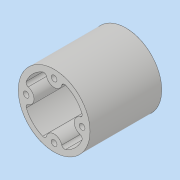
# Autodesk Inventor part: SpoolSmall
Saved by Autodesk Inventor 2017 (Build 210142000, 142)
## iProperties
Created: 2018-04-03
Part Number: SpoolSmall
Material: Generic
Document SubType Name: Modeling
Designer: Derek Wider
Density: 1 g/cm^3
Appearance: Default
Author: Derek Wider
Autodesk Inventor part; units mm, degrees
ref_plane "YZ Plane" through (0, 0, 0) normal (1, 0, 0) x (0, 1, 0)
ref_plane "XZ Plane" through (0, 0, 0) normal (0, 1, 0) x (-1, 0, 0)
ref_plane "XY Plane" through (0, 0, 0) normal (0, 0, 1) x (1, 0, 0)
sketch "Sketch1" plane through (0, 0, 0) normal (0, 0, 1) x (1, 0, 0)
  circle A0 centre (0, 0) radius 15.875
  dimension "d0" = 31.75
  constraints: 1 centre point, 1 coincident
  measures "d0" diameter of A0
extrude "Extrusion1" add sketch "Sketch1" along normal blind 31.75
shell "Shell1" thickness 2.54 removed faces 2 at (-8.4384, -2.4592, 31.75) at (-8.4384, -2.4592, 0)
sketch "Sketch3" plane through (0, 0, 31.75) normal (0, 0, 1) x (1, 0, 0)
  circle A0 centre (0, 12.3825) radius 1.27
  circle A1 centre (0, 12.3825) radius 3.4925
  circle A2 centre (0, 0) radius 15.875 projected
  dimension "d4" = 2.54
  dimension "d5" = 6.985
  constraints: 2 centre point, 1 coincident, 1 tangent
  measures "d4" diameter of A0
  measures "d5" diameter of A1
extrude "Extrusion2" cut sketch "Sketch3" against normal up to surface (31.75 mm away) contours A0
extrude "Extrusion3" add sketch "Sketch3" against normal up to surface (31.75 mm away) contours A1
fillet "Fillet1" radius 1.27 2 edges at (-3.457, 12.8791, 15.875) (3.457, 12.8791, 15.875)
pattern_circular "Circular Pattern2" count 4 over 360 about axis through (0, 0, 0) along (0, 0, 1) of "Extrusion3", "Fillet1", "Extrusion2"
body "Solid1"
